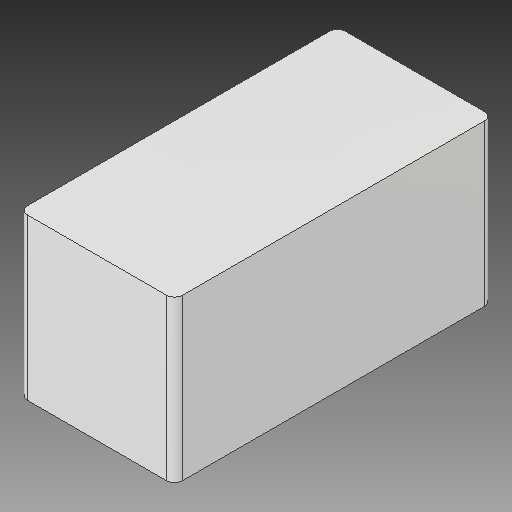
# Autodesk Inventor part: Medio
Saved by Autodesk Inventor 2019 (Build 230136000, 136)
## iProperties
Created: 2016-09-26
Part Number: Medio
Material: Plástico ABS
Document SubType Name: Modeling
Designer: Julian
Density: 1.06 g/cm^3
Appearance: Suave - Blanco
Mass: 17.4497 g
Surface Area: 40.4725 cm^2
Volume: 16.4619 cm^3
Author: Julian
Autodesk Inventor part; units mm, degrees
ref_plane "YZ Plane" through (0, 0, 0) normal (1, 0, 0) x (0, 1, 0)
ref_plane "XZ Plane" through (0, 0, 0) normal (0, 1, 0) x (-1, 0, 0)
ref_plane "XY Plane" through (0, 0, 0) normal (0, 0, 1) x (1, 0, 0)
sketch "Boceto1" plane through (0, 0, 0) normal (0, 1, 0) x (-1, 0, 0)
  line L0 (9.9, 20.3) -> (-9.9, 20.3)
  line L1 (-9.9, 20.3) -> (-9.9, -20.3)
  line L2 (-9.9, -20.3) -> (9.9, -20.3)
  line L3 (9.9, -20.3) -> (9.9, 20.3)
  line L4 (9.9, 20.3) -> (-9.9, -20.3) construction
  line L5 (-9.9, 20.3) -> (9.9, -20.3) construction
  point P0 (0, 0)
  dimension "d0" = 19.8
  dimension "d1" = 40.6
  constraints: 12 end point, 2 midpoint, 2 parallel, 1 horizontal, 1 perpendicular
  measures "d0" distance of L2.end L1.end
  measures "d1" distance of L1.end L0.end
extrude "Extrusión1" add sketch "Boceto1" against normal blind 20.5
fillet "Empalme1" radius 1 4 edges at (9.9, -10.25, 20.3) (-9.9, -10.25, 20.3) (9.9, -10.25, -20.3) (-9.9, -10.25, -20.3)
